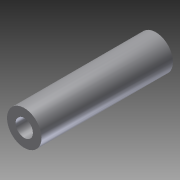
# Autodesk Inventor part: Distance Limiter
Saved by Autodesk Inventor 2012 (Build 160160000, 160)
## iProperties
Created: 2013-01-19
Part Number: Distance Limiter
Material: Default
Document SubType Name: Modeling
Designer: William
Density: 1 g/cm^3
Author: William
Autodesk Inventor part; units mm, degrees
ref_plane "YZ Plane" through (0, 0, 0) normal (1, 0, 0) x (0, 1, 0)
ref_plane "XZ Plane" through (0, 0, 0) normal (0, 1, 0) x (-1, 0, 0)
ref_plane "XY Plane" through (0, 0, 0) normal (0, 0, 1) x (1, 0, 0)
sketch "Sketch1" plane through (0, 0, 0) normal (0, 0, 1) x (1, 0, 0)
  circle A0 centre (5.2764, 0) radius 5
  circle A1 centre (5.2764, 0) radius 2.5146
  point P0 (0, 0)
  dimension "d0" = 10
  dimension "d1" = 5.0292
  constraints: 2 centre point, 1 coincident
  measures "d0" diameter of A0
  measures "d1" diameter of A1
extrude "Extrusion1" add sketch "Sketch1" along normal blind 38.1
body "Solid1"
